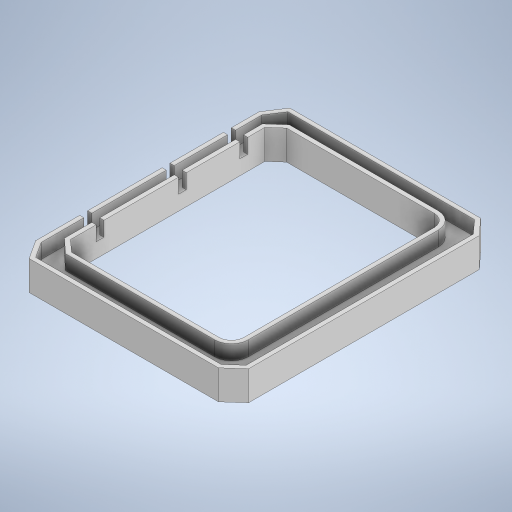
# Autodesk Inventor part: Robotic_Template_Tray
Saved by Autodesk Inventor 2023 (Build 270158000, 158)
## iProperties
Created: 2023-03-10
Part Number: Robotic_Template_Tray
Material: Generic
Document SubType Name: Modeling
Designer: 1senadi
Density: 1 g/cm^3
Appearance: Default
Author: 1senadi
Autodesk Inventor part; units mm, degrees
ref_plane "YZ Plane" through (0, 0, 0) normal (1, 0, 0) x (0, 1, 0)
ref_plane "XZ Plane" through (0, 0, 0) normal (0, 1, 0) x (-1, 0, 0)
sketch "Sketch1" plane through (0, 0, 0) normal (0, 1, 0) x (-1, 0, 0)
  line L0 (0, 0) -> (68.89, 0)
  line L1 (68.89, 0) -> (68.89, -86.42)
  line L2 (68.89, -86.42) -> (0, -86.42)
  line L3 (0, -86.42) -> (0, 0)
  line L4 (68.89, 0) -> (75.48, 0)
  line L5 (75.48, 0) -> (75.48, -86.42)
  line L6 (75.48, -86.42) -> (68.89, -86.42)
  line L7 (0, -86.42) -> (0, -94.04)
  line L8 (0, -94.04) -> (75.48, -94.04)
  line L9 (75.48, -94.04) -> (75.48, -86.42)
  line L10 (0, 0) -> (-11.84, 0)
  line L11 (-11.84, 0) -> (-11.84, -94.04)
  line L12 (-11.84, -94.04) -> (0, -94.04)
  line L13 (68.89, 0) -> (68.89, 10.69)
  line L14 (68.89, 10.69) -> (-11.84, 10.69)
  line L15 (-11.84, 10.69) -> (-11.84, 0)
  line L16 (68.89, 10.69) -> (75.48, 10.69)
  line L17 (75.48, 10.69) -> (75.48, 0)
  dimension "d0" = 68.89
  dimension "d1" = 86.42
  dimension "d2" = 6.59
  dimension "d3" = 7.62
  dimension "d4" = 11.84
  dimension "d5" = 10.69
  constraints: 36 end point, 9 perpendicular, 2 collinear, 2 horizontal, 2 parallel, 2 point on line, 2 vertical
  measures "d0" distance of L1.end L2.end
  measures "d1" distance of L0.end L1.end
  measures "d2" distance of L0.end L4.end
  measures "d3" distance of L2.end L7.end
  measures "d4" distance of L0.start L10.end
  measures "d5" distance of L0.end L13.end
extrude "Extrusion1" add sketch "Sketch1" along normal blind 11.83 contours L10 L15 L14 L13 L0 | L3 L7 L12 L11 L10 | L4 L5 L6 L1 | L13 L16 L17 L4 | L2 L6 L9 L8 L7
sketch "Sketch2" plane through (0, 11.83, 0) normal (0, 1, 0) x (1, 0, 0)
  line L0 (-68.89, 86.42) -> (-68.89, 94.04)
  line L1 (11.84, 94.04) -> (-75.48, 94.04) projected
  line L2 (-68.89, 94.04) -> (-68.89, 75.38)
  line L3 (-68.89, 0) -> (-68.89, 86.42) projected
  line L4 (-75.48, 94.04) -> (-75.48, -10.69) projected
  line L5 (-68.89, 75.38) -> (-75.48, 75.38)
  line L6 (-75.48, 75.38) -> (-75.48, 72.25)
  line L7 (-75.48, 75.38) -> (-72.35, 75.38) construction
  line L8 (-75.48, 72.25) -> (-68.89, 72.25)
  line L9 (-68.89, 75.38) -> (-68.89, 72.25)
  line L10 (-68.89, 94.04) -> (-68.89, 50.73)
  line L11 (-68.89, 50.73) -> (-75.48, 50.73)
  line L12 (-75.48, 50.73) -> (-75.48, 47.6)
  line L13 (-75.48, 47.6) -> (-68.89, 47.6)
  line L14 (-68.89, 50.73) -> (-68.89, 47.6)
  line L15 (-68.89, 94.04) -> (-68.89, 17.63)
  line L16 (-68.89, 17.63) -> (-75.48, 17.63)
  line L17 (-75.48, 17.63) -> (-75.48, 14.5)
  line L18 (-75.48, 14.5) -> (-68.89, 14.5)
  line L19 (-68.89, 17.63) -> (-68.89, 14.5)
  point P0 (0, 0)
  dimension "d8" = 18.66
  dimension "d10" = 3.13
  dimension "d11" = 90
  dimension "d12" = 43.31
  dimension "d13" = 3.13
  dimension "d14" = 76.41
  dimension "d15" = 3.13
  constraints: 34 end point, 12 point on line, 9 perpendicular, 2 collinear, 1 horizontal, 1 vertical
  measures "d8" distance of L0.end L2.end
  measures "d10" distance of L5.end L6.end
  measures "d11" angle of L6 L7
  measures "d12" distance of L0.end L10.end
  measures "d13" distance of L11.end L12.end
  measures "d14" distance of L0.end L15.end
  measures "d15" distance of L16.end L17.end
extrude "Extrusion2" cut sketch "Sketch2" against normal blind 7.26 contours L3 L8 L4 L5 | L3 L13 L4 L11 | L3 L18 L4 L16
fillet "Fillet1" radius 5 2 edges at (0, 5.915, -86.42) (0, 5.915, 0)
chamfer "Chamfer1" distance 4.17 distance2 4.63 2 edges at (-68.89, 5.915, -86.42) (-68.89, 5.915, 0) measured on face at (-68.89, 1.5233, -34.6833)
chamfer "Chamfer2" distance 4.87 distance2 7.5 1 edges at (-75.48, 5.915, -94.04) measured on face at (-17.2667, 7.8867, -94.04)
chamfer "Chamfer3" distance 7.5 distance2 4.87 1 edges at (-75.48, 5.915, 10.69) measured on face at (-75.48, 1.5233, -49.3667)
chamfer "Chamfer5" distance 6.36 distance2 5.73 1 edges at (11.84, 5.915, 10.69) measured on face at (-43.1267, 3.9433, 10.69)
chamfer "Chamfer6" distance 6.36 distance2 5.73 1 edges at (11.84, 5.915, -94.04) measured on face at (11.84, 3.9433, -28.04)
sketch "Sketch3" plane through (0, 0, 0) normal (0, -1, 0) x (1, 0, 0)
  line L0 (5.48, 10.69) -> (11.84, 4.96) projected
  line L1 (-70.61, 10.69) -> (5.48, 10.69) projected
  line L2 (-75.48, 3.19) -> (-70.61, 10.69) projected
  line L3 (-75.48, -86.54) -> (-75.48, 3.19) projected
  line L4 (-70.61, -94.04) -> (-75.48, -86.54) projected
  line L5 (6.11, -94.04) -> (-70.61, -94.04) projected
  line L6 (11.84, 4.96) -> (11.84, -87.68) projected
  arc A0 (-5, -86.42) -> (0, -81.42) centre (-5, -81.42) ccw projected
  line L7 (-64.26, -86.42) -> (-5, -86.42) projected
  line L8 (-68.89, -82.25) -> (-64.26, -86.42) projected
  line L9 (-68.89, -4.17) -> (-68.89, -82.25) projected
  line L10 (-5, 0) -> (-64.26, 0) projected
  arc A1 (0, -5) -> (-5, 0) centre (-5, -5) ccw projected
  line L11 (0, -81.42) -> (0, -5) projected
  line L12 (4.8271, 8.99) -> (10.14, 4.2034)
  line L13 (10.14, 4.2034) -> (10.14, -87.0271)
  line L14 (8.6349, -90.5535) -> (8.3777, -90.86)
  line L15 (5.3534, -92.34) -> (-69.6869, -92.34)
  line L16 (-69.6869, -92.34) -> (-73.78, -86.0365)
  line L17 (-73.78, -86.0365) -> (-73.78, 2.6865)
  line L18 (-73.78, 2.6865) -> (-69.6869, 8.99)
  line L19 (-69.6869, 8.99) -> (4.8271, 8.99)
  line L20 (-67.5942, 1.7) -> (-70.59, -1.2958)
  line L21 (-70.59, -1.2958) -> (-70.59, -83.0068)
  line L22 (-70.59, -83.0068) -> (-64.9127, -88.12)
  line L23 (-64.9127, -88.12) -> (-5, -88.12)
  arc A2 (-5, -88.12) -> (1.7, -81.42) centre (-5, -81.42) ccw
  line L24 (1.7, -81.42) -> (1.7, -5)
  arc A3 (1.7, -5) -> (-5, 1.7) centre (-5, -5) ccw
  line L25 (-5, 1.7) -> (-67.5942, 1.7)
  line L26 (11.84, -87.68) -> (6.11, -94.04) projected
  line L27 (6.11, -94.04) -> (11.84, -87.68) projected
  line L28 (8.975, -90.86) -> (10.675, -90.86) construction
  line L29 (8.975, -90.86) -> (7.712, -89.7221)
  line L30 (7.712, -89.7221) -> (5.3534, -92.34)
  line L31 (7.712, -89.7221) -> (10.14, -87.0271)
  line L32 (-64.26, 0) -> (-68.89, -4.17) projected
  line L33 (-66.696, -2.194) -> (-67.8337, -0.9308)
  line L34 (-67.8337, -0.9308) -> (-64.9127, 1.7)
  line L35 (-67.8337, -0.9308) -> (-70.59, -3.4132)
  point P0 (0, 0)
  dimension "d34" = 1.7
  dimension "d35" = 1.7
  dimension "d50" = 1.7
  dimension "d51" = 1.7
  constraints: 42 end point, 7 point on line, 4 point on circle, 3 perpendicular, 2 centre point, 1 horizontal, 1 midpoint, 9 other
  measures "d34" distance between parallel lines of L1 L19
  measures "d35" distance between parallel lines of L10 L25
  measures "d50" distance of L28.start L29.end
  measures "d51" distance of L33.start L33.end
extrude "Extrusion3" cut sketch "Sketch3" against normal up to surface (11.83 mm away) contours L7 L8 L9 L32 L10 A1 L11 A0 | L12 L13 L31 L30 L15 L16 L17 L18 L19 | L25 L34 L35 L21 L20
ref_plane "Work Plane1" through (0, 5.93, 0) normal (0, 1, 0) x (1, 0, 0)
sketch "Sketch4" plane through (0, 5.93, 0) normal (0, 1, 0) x (1, 0, 0)
  line L0 (-70.59, 14.5) -> (-70.59, 3.4132) projected
  line L1 (-64.9127, -1.7) -> (-5, -1.7) projected
  arc A0 (-5, -1.7) -> (1.7, 5) centre (-5, 5) ccw projected
  line L2 (1.7, 5) -> (1.7, 81.42) projected
  arc A1 (1.7, 81.42) -> (-5, 88.12) centre (-5, 81.42) ccw projected
  line L3 (-5, 88.12) -> (-64.9127, 88.12) projected
  line L4 (-64.9127, 88.12) -> (-70.59, 83.0068) projected
  line L5 (-70.59, 83.0068) -> (-70.59, 75.38) projected
  line L6 (-70.59, 75.38) -> (-68.89, 75.38) projected
  line L7 (-68.89, 75.38) -> (-68.89, 82.25) projected
  line L8 (-64.26, 86.42) -> (-68.89, 82.25) projected
  line L9 (-64.26, 86.42) -> (-5, 86.42) projected
  arc A2 (0, 81.42) -> (-5, 86.42) centre (-5, 81.42) ccw projected
  line L10 (0, 81.42) -> (0, 5) projected
  arc A3 (-5, 0) -> (0, 5) centre (-5, 5) ccw projected
  line L11 (-5, 0) -> (-64.26, 0) projected
  line L12 (-68.89, 4.17) -> (-68.89, 14.5) projected
  line L13 (-68.89, 14.5) -> (-70.59, 14.5) projected
  line L14 (-73.78, -2.6865) -> (-73.78, 14.5) projected
  line L15 (-73.78, 14.5) -> (-75.48, 14.5) projected
  line L16 (-75.48, 14.5) -> (-75.48, -3.19) projected
  line L17 (-70.61, -10.69) -> (-75.48, -3.19) projected
  line L18 (-70.61, -10.69) -> (5.48, -10.69) projected
  line L19 (11.84, -4.96) -> (5.48, -10.69) projected
  line L20 (11.84, -4.96) -> (11.84, 87.68) projected
  line L21 (6.11, 94.04) -> (-70.61, 94.04) projected
  line L22 (-75.48, 86.54) -> (-70.61, 94.04) projected
  line L23 (-75.48, 86.54) -> (-75.48, 75.38) projected
  line L24 (-75.48, 75.38) -> (-73.78, 75.38) projected
  line L25 (-73.78, 75.38) -> (-73.78, 86.0365) projected
  line L26 (-73.78, 86.0365) -> (-69.6869, 92.34) projected
  line L27 (-69.6869, 92.34) -> (5.3534, 92.34) projected
  line L28 (10.14, 87.0271) -> (10.14, -4.2034) projected
  line L29 (10.14, -4.2034) -> (4.8271, -8.99) projected
  line L30 (4.8271, -8.99) -> (-69.6869, -8.99) projected
  line L31 (-69.6869, -8.99) -> (-73.78, -2.6865) projected
  line L32 (-70.59, 17.63) -> (-70.59, 14.5) projected
  line L33 (-68.89, 14.5) -> (-70.59, 14.5) projected
  line L34 (-68.89, 17.63) -> (-68.89, 14.5) projected
  line L35 (-70.59, 17.63) -> (-68.89, 17.63) projected
  line L36 (-70.59, 50.73) -> (-70.59, 47.6) projected
  line L37 (-68.89, 47.6) -> (-70.59, 47.6) projected
  line L38 (-68.89, 50.73) -> (-68.89, 47.6) projected
  line L39 (-70.59, 50.73) -> (-68.89, 50.73) projected
  line L40 (-70.59, 75.38) -> (-70.59, 72.25) projected
  line L41 (-68.89, 72.25) -> (-70.59, 72.25) projected
  line L42 (-68.89, 75.38) -> (-68.89, 72.25) projected
  line L43 (-70.59, 75.38) -> (-68.89, 75.38) projected
  line L44 (-73.78, 72.25) -> (-73.78, 75.38) projected
  line L45 (-75.48, 75.38) -> (-73.78, 75.38) projected
  line L46 (-75.48, 72.25) -> (-75.48, 75.38) projected
  line L47 (-73.78, 72.25) -> (-75.48, 72.25) projected
  line L48 (-73.78, 47.6) -> (-73.78, 50.73) projected
  line L49 (-75.48, 50.73) -> (-73.78, 50.73) projected
  line L50 (-75.48, 47.6) -> (-75.48, 50.73) projected
  line L51 (-73.78, 47.6) -> (-75.48, 47.6) projected
  line L52 (-73.78, 14.5) -> (-73.78, 17.63) projected
  line L53 (-75.48, 17.63) -> (-73.78, 17.63) projected
  line L54 (-75.48, 14.5) -> (-75.48, 17.63) projected
  line L55 (-73.78, 14.5) -> (-75.48, 14.5) projected
  arc A4 (0, 81.42) -> (-5, 86.42) centre (-5, 81.42) ccw projected
  line L56 (-64.26, 86.42) -> (-5, 86.42) projected
  line L57 (-68.89, 82.25) -> (-64.26, 86.42) projected
  line L58 (-68.89, 4.17) -> (-68.89, 82.25) projected
  line L59 (-5, 0) -> (-64.26, 0) projected
  arc A5 (-5, 0) -> (0, 5) centre (-5, 5) ccw projected
  line L60 (0, 81.42) -> (0, 5) projected
  line L61 (-64.9127, 88.12) -> (-5, 88.12) projected
  arc A6 (1.7, 81.42) -> (-5, 88.12) centre (-5, 81.42) ccw projected
  line L62 (1.7, 81.42) -> (1.7, 5) projected
  arc A7 (-5, -1.7) -> (1.7, 5) centre (-5, 5) ccw projected
  line L63 (-5, -1.7) -> (-64.9127, -1.7) projected
  line L64 (-70.59, 3.4132) -> (-70.59, 83.0068) projected
  line L65 (-70.59, 83.0068) -> (-64.9127, 88.12) projected
  line L66 (5.3534, 92.34) -> (-69.6869, 92.34) projected
  line L67 (-69.6869, 92.34) -> (-73.78, 86.0365) projected
  line L68 (-73.78, 86.0365) -> (-73.78, -2.6865) projected
  line L69 (-73.78, -2.6865) -> (-69.6869, -8.99) projected
  line L70 (-69.6869, -8.99) -> (4.8271, -8.99) projected
  line L71 (4.8271, -8.99) -> (10.14, -4.2034) projected
  line L72 (10.14, -4.2034) -> (10.14, 87.0271) projected
  line L73 (5.48, -10.69) -> (11.84, -4.96) projected
  line L74 (-70.61, -10.69) -> (5.48, -10.69) projected
  line L75 (-75.48, -3.19) -> (-70.61, -10.69) projected
  line L76 (-75.48, 86.54) -> (-75.48, -3.19) projected
  line L77 (-70.61, 94.04) -> (-75.48, 86.54) projected
  line L78 (6.11, 94.04) -> (-70.61, 94.04) projected
  line L79 (11.84, -4.96) -> (11.84, 87.68) projected
  line L80 (-70.59, 72.25) -> (-70.59, 50.73) projected
  line L81 (-70.59, 50.73) -> (-68.89, 50.73) projected
  line L82 (-68.89, 50.73) -> (-68.89, 72.25) projected
  line L83 (-68.89, 72.25) -> (-70.59, 72.25) projected
  line L84 (-70.59, 47.6) -> (-70.59, 17.63) projected
  line L85 (-70.59, 17.63) -> (-68.89, 17.63) projected
  line L86 (-68.89, 17.63) -> (-68.89, 47.6) projected
  line L87 (-68.89, 47.6) -> (-70.59, 47.6) projected
  line L88 (7.1358, 92.34) -> (10.14, 89.3358) projected
  line L89 (10.14, 89.3358) -> (7.1358, 92.34) projected
  line L90 (11.84, 87.68) -> (6.11, 94.04) projected
  line L91 (6.11, 94.04) -> (11.84, 87.68) projected
  line L92 (10.14, 87.0271) -> (5.3534, 92.34) projected
  line L93 (5.3534, 92.34) -> (10.14, 87.0271) projected
  line L94 (-64.26, 0) -> (-68.89, 4.17) projected
  line L95 (-68.89, 4.17) -> (-64.26, 0) projected
  line L96 (-64.9127, -1.7) -> (-70.59, 3.4132) projected
  line L97 (-70.59, 3.4132) -> (-64.9127, -1.7) projected
  point P0 (0, 0)
  point P1 (-73.78, 47.6)
  point P2 (-73.78, 17.63)
  point P3 (-73.78, 14.5)
  point P4 (-73.78, 75.38)
  point P5 (-73.78, 72.25)
  point P6 (-73.78, 50.73)
  point P7 (-70.59, 50.73)
  point P8 (-70.59, 72.25)
  point P9 (-70.59, 75.38)
  point P10 (-70.59, 14.5)
  point P11 (-70.59, 17.63)
  point P12 (-70.59, 47.6)
extrude "Extrusion4" add sketch "Sketch4" against normal blind 2.08 contours L13 L12 L94 L11 A3 L10 A2 L9 L8 L7 L6 L5 L4 L3 A1 L2 A0 L1 L96 L0 | L32 L35 L34 L13 | L34 L58 L38 L42 L7 L8 L9 A2 L10 A3 L11 L94 L12 | L64 L37 L58 L35 | L36 L39 L38 L37 | L64 L41 L58 L39 | L40 L6 L42 L41 | L14 L52 L68 L48 L44 L25 L26 L27 L92 L28 L29 L30 L31
sketch "Sketch6" plane through (0, 5.93, 0) normal (0, 1, 0) x (1, 0, 0)
  line L0 (5.3534, 92.34) -> (10.14, 87.0271) projected
  line L1 (-69.6869, 92.34) -> (5.3534, 92.34) projected
  line L2 (-73.78, 86.0365) -> (-69.6869, 92.34) projected
  line L3 (-73.78, 75.38) -> (-73.78, 86.0365) projected
  line L4 (-73.78, 75.38) -> (-73.78, 72.25) projected
  line L5 (-73.78, 50.73) -> (-73.78, 72.25) projected
  line L6 (-73.78, 50.73) -> (-73.78, 47.6) projected
  line L7 (-73.78, 17.63) -> (-73.78, 47.6) projected
  line L8 (-73.78, 17.63) -> (-73.78, 14.5) projected
  line L9 (-73.78, -2.6865) -> (-73.78, 14.5) projected
  line L10 (-69.6869, -8.99) -> (-73.78, -2.6865) projected
  line L11 (4.8271, -8.99) -> (-69.6869, -8.99) projected
  line L12 (10.14, -4.2034) -> (4.8271, -8.99) projected
  line L13 (10.14, 87.0271) -> (10.14, -4.2034) projected
  arc A0 (-5, 0) -> (0, 5) centre (-5, 5) ccw projected
  line L14 (0, 81.42) -> (0, 5) projected
  arc A1 (0, 81.42) -> (-5, 86.42) centre (-5, 81.42) ccw projected
  line L15 (-64.26, 86.42) -> (-5, 86.42) projected
  line L16 (-68.89, 82.25) -> (-64.26, 86.42) projected
  line L17 (-68.89, 75.38) -> (-68.89, 82.25) projected
  line L18 (-70.59, 75.38) -> (-68.89, 75.38) projected
  line L19 (-70.59, 83.0068) -> (-70.59, 75.38) projected
  line L20 (-64.9127, 88.12) -> (-70.59, 83.0068) projected
  line L21 (-5, 88.12) -> (-64.9127, 88.12) projected
  arc A2 (1.7, 81.42) -> (-5, 88.12) centre (-5, 81.42) ccw projected
  line L22 (1.7, 5) -> (1.7, 81.42) projected
  arc A3 (-5, -1.7) -> (1.7, 5) centre (-5, 5) ccw projected
  line L23 (-64.9127, -1.7) -> (-5, -1.7) projected
  line L24 (-70.59, 3.4132) -> (-64.9127, -1.7) projected
  line L25 (-70.59, 14.5) -> (-70.59, 3.4132) projected
  line L26 (-68.89, 14.5) -> (-70.59, 14.5) projected
  line L27 (-68.89, 4.17) -> (-68.89, 14.5) projected
  line L28 (-64.26, 0) -> (-68.89, 4.17) projected
  line L29 (-5, 0) -> (-64.26, 0) projected
  line L30 (-70.59, 47.6) -> (-70.59, 17.63) projected
  line L31 (-68.89, 47.6) -> (-70.59, 47.6) projected
  line L32 (-68.89, 17.63) -> (-68.89, 47.6) projected
  line L33 (-70.59, 17.63) -> (-68.89, 17.63) projected
  line L34 (-70.59, 72.25) -> (-70.59, 50.73) projected
  line L35 (-68.89, 72.25) -> (-70.59, 72.25) projected
  line L36 (-68.89, 50.73) -> (-68.89, 72.25) projected
  line L37 (-70.59, 50.73) -> (-68.89, 50.73) projected
  line L38 (-68.89, 14.5) -> (-68.89, 17.63)
  line L39 (-68.89, 4.17) -> (-68.89, 82.25) projected
  line L40 (-68.89, 75.38) -> (-68.89, 72.25)
  line L41 (-68.89, 50.73) -> (-68.89, 47.6)
  point P0 (0, 0)
  constraints: 6 end point, 3 collinear
extrude "Extrusion5" cut sketch "Sketch6" against normal up to surface (2.08 mm away) contours L29 L28 L27 L38 L32 L39 L36 L17 L16 L15 A1 L14 A0
body "Solid1"
